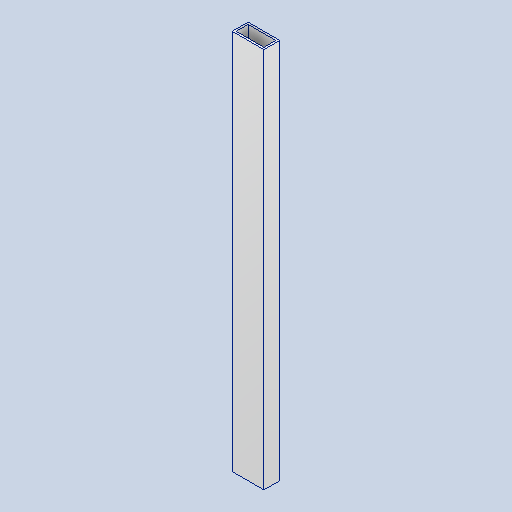
# Autodesk Inventor part: sideExtrusion
Saved by Autodesk Inventor 2022.2 (Build 262287000, 287)
## iProperties
Created: 2022-01-19
Part Number: sideExtrusion
Material: Aluminum 6061
Document SubType Name: Modeling
Designer: robst
Density: 2.7 g/cm^3
Appearance: Aluminum - Flat
Author: robst
Autodesk Inventor part; units mm, degrees
ref_plane "YZ Plane" through (0, 0, 0) normal (1, 0, 0) x (0, 1, 0)
ref_plane "XZ Plane" through (0, 0, 0) normal (0, 1, 0) x (-1, 0, 0)
ref_plane "XY Plane" through (0, 0, 0) normal (0, 0, 1) x (1, 0, 0)
sketch "Sketch1" plane through (0, 0, 0) normal (0, 0, 1) x (1, 0, 0)
  line L0 (-25.4, -304.8) -> (25.4, -304.8)
  line L1 (25.4, -304.8) -> (25.4, 304.8)
  line L2 (25.4, 304.8) -> (-25.4, 304.8)
  line L3 (-25.4, 304.8) -> (-25.4, -304.8)
  line L4 (-25.4, -304.8) -> (25.4, 304.8) construction
  line L5 (25.4, -304.8) -> (-25.4, 304.8) construction
  point P0 (0, 0)
  dimension "d0" = 50.8
  dimension "d1" = 609.6
  constraints: 12 end point, 2 midpoint, 2 parallel, 1 horizontal, 1 perpendicular
  measures "d0" distance of L0.start L0.end
  measures "d1" distance of L1.end L0.end
extrude "Extrusion1" add sketch "Sketch1" along normal mid plane 25.4
sketch "Sketch2" plane through (0, 0, 0) normal (0, 1, 0) x (-1, 0, 0)
  line L0 (-22.225, 9.525) -> (-22.225, -9.525)
  line L1 (-22.225, -9.525) -> (22.225, -9.525)
  line L2 (22.225, -9.525) -> (22.225, 9.525)
  line L3 (22.225, 9.525) -> (-22.225, 9.525)
  line L4 (-22.225, 9.525) -> (22.225, -9.525) construction
  line L5 (-22.225, -9.525) -> (22.225, 9.525) construction
  line L6 (25.4, -12.7) -> (25.4, 12.7) projected
  line L7 (25.4, 12.7) -> (-25.4, 12.7) projected
  point P0 (0, 0)
  dimension "d4" = 3.175
  dimension "d5" = 3.175
  constraints: 12 end point, 2 midpoint, 2 parallel, 1 perpendicular, 1 vertical
  measures "d4" distance between parallel lines of L2 L6
  measures "d5" distance between parallel lines of L7 L3
extrude "Extrusion2" cut sketch "Sketch2" along normal through all both and the other way through all
equation "\"d0\" = width"
equation "\"d1\" = height"
equation "\"d2\" = depth"
equation "\"d4\" = wallThickness"
equation "\"d5\" = wallThickness"
equation "\"depth\" = 25.4"
equation "\"width\" = 50.8"
equation "\"height\" = 609.6"
equation "\"wallThickness\" = 3.175"
body "Solid1"
